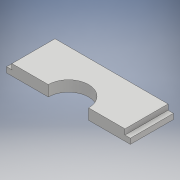
# Autodesk Inventor part: Lid
Saved by Autodesk Inventor 2018 (Build 220112000, 112)
## iProperties
Created: 2019-07-19
Part Number: Lid
Material: Generic
Document SubType Name: Modeling
Designer: aal_9
Density: 1 g/cm^3
Appearance: Default
Author: aal_9
Autodesk Inventor part; units mm, degrees
ref_plane "YZ Plane" through (0, 0, 0) normal (1, 0, 0) x (0, 1, 0)
ref_plane "XZ Plane" through (0, 0, 0) normal (0, 1, 0) x (-1, 0, 0)
ref_plane "XY Plane" through (0, 0, 0) normal (0, 0, 1) x (1, 0, 0)
sketch "Sketch1" plane through (0, 0, 0) normal (0, 1, 0) x (-1, 0, 0)
  line L0 (21, 2) -> (-21, 2)
  line L1 (-21, 2) -> (-21, -2)
  line L2 (-21, -2) -> (21, -2)
  line L3 (21, -2) -> (21, 2)
  line L4 (23, 0) -> (-23, 0)
  line L5 (-23, 0) -> (-23, -2)
  line L6 (-23, -2) -> (23, -2)
  line L7 (23, -2) -> (23, 0)
  point P0 (0, 0)
  dimension "d0" = 42
  dimension "d1" = 4
  dimension "d2" = 21
  dimension "d3" = 2
  dimension "d4" = 2
  dimension "d5" = 46
  dimension "d6" = 2
  dimension "d7" = 2
  constraints: 16 end point, 4 parallel, 2 horizontal, 2 perpendicular
  measures "d0" distance of L2.end L1.end
  measures "d1" distance of L1.end L0.end
  measures "d2" distance from line of point (0, 0) L3
  measures "d3" distance from line of L2 point (0, 0)
  measures "d4" distance between parallel lines of L7 L3
  measures "d5" distance of L5.end L6.end
  measures "d6" distance between parallel lines of L0 L4
  measures "d7" distance between parallel lines of L4 L6
extrude "Extrusion1" add sketch "Sketch1" along normal blind 16
sketch "Sketch2" plane through (-21, 0, 2) normal (0, 0, 1) x (1, 0, 0)
  circle A0 centre (21, 0) radius 7.5
  dimension "d10" = 15
  constraints: 1 centre point, 1 coincident
  measures "d10" diameter of A0
extrude "Extrusion2" cut sketch "Sketch2" against normal up to next
equation "\"d2\" = 0.5 * d0"
equation "\"d3\" = 0.5 * d1"
body "Solid1"
